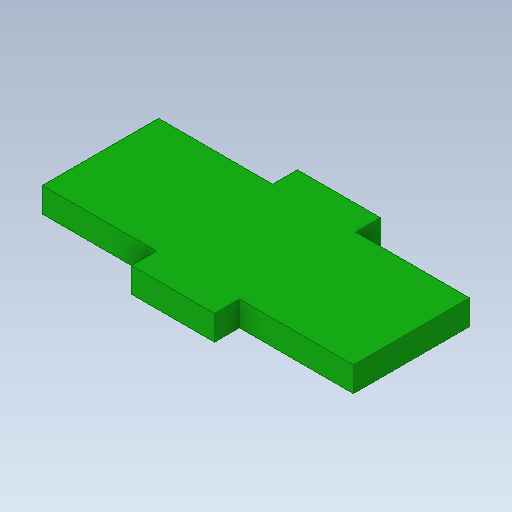
# Autodesk Inventor part: Top1
Saved by Autodesk Inventor 2020 (Build 240168000, 168)
## iProperties
Created: 2020-03-13
Part Number: Top1
Material: Genérico
Document SubType Name: Modeling
Designer: joser
Density: 1 g/cm^3
Appearance: Verde oscuro
Author: joser
Autodesk Inventor part; units mm, degrees
ref_plane "YZ Plane" through (0, 0, 0) normal (1, 0, 0) x (0, 1, 0)
ref_plane "XZ Plane" through (0, 0, 0) normal (0, 1, 0) x (-1, 0, 0)
ref_plane "XY Plane" through (0, 0, 0) normal (0, 0, 1) x (1, 0, 0)
sketch "Boceto1" plane through (0, 0, 0) normal (0, 1, 0) x (-1, 0, 0)
  line L0 (0, 0) -> (-10, 0)
  line L1 (-23.7525, -3) -> (-23.7525, -17)
  line L2 (-10, -20) -> (0, -20)
  line L3 (13.7525, -17) -> (13.7525, -3)
  line L4 (0, -17) -> (0, -20)
  line L5 (-10, -17) -> (-10, -20)
  line L6 (-23.7525, -17) -> (-10, -17)
  line L7 (0, -17) -> (13.7525, -17)
  line L8 (0, -3) -> (0, 0)
  line L9 (-10, -3) -> (-10, 0)
  line L10 (13.7525, -3) -> (0, -3)
  line L11 (-10, -3) -> (-23.7525, -3)
  dimension "d0" = 37.505
  dimension "d3" = 20
  dimension "d4" = 10
  dimension "d5" = 3
  constraints: 24 end point, 6 parallel, 4 equal length, 3 horizontal, 3 perpendicular, 2 collinear, 2 vertical, 1 coincident
  measures "d0" distance between parallel lines of L1 L3
  measures "d3" distance between parallel lines of L2 L0
  measures "d4" distance between parallel lines of L5 L4
  measures "d5" distance between parallel lines of L2 L7
extrude "Extrusión1" add sketch "Boceto1" along normal blind 3
